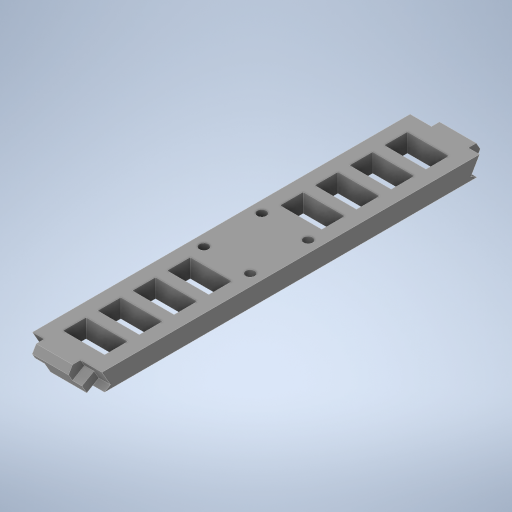
# Autodesk Inventor part: base
Saved by Autodesk Inventor 2024.3 (Build 283343000, 343)
## iProperties
Created: 2024-10-09
Part Number: base
Material: Generic
Document SubType Name: Modeling
Designer: pjcaa
Density: 1 g/cm^3
Appearance: Default(2)
Author: pjcaa
Autodesk Inventor part; units mm, degrees
ref_plane "YZ Plane" through (0, 0, 0) normal (1, 0, 0) x (0, 1, 0)
ref_plane "XZ Plane" through (0, 0, 0) normal (0, 1, 0) x (-1, 0, 0)
ref_plane "XY Plane" through (0, 0, 0) normal (0, 0, 1) x (1, 0, 0)
sketch "Sketch1" plane through (0, 0, 0) normal (0, 0, 1) x (1, 0, 0)
  line L0 (-85, -15) -> (85, -15)
  line L1 (85, -15) -> (85, 15)
  line L2 (85, 15) -> (-85, 15)
  line L3 (-85, 15) -> (-85, -15)
  line L4 (-85, -15) -> (85, 15) construction
  line L5 (85, -15) -> (-85, 15) construction
  point P0 (0, 0)
  dimension "d0" = 170
  dimension "d1" = 30
  constraints: 12 end point, 2 midpoint, 2 parallel, 1 horizontal, 1 perpendicular
  measures "d0" distance of L2.end L1.end
  measures "d1" distance of L1.end L0.end
extrude "Extrusion1" add sketch "Sketch1" along normal blind 8
sketch "Sketch2" plane through (-85, 15, 0) normal (0, 1, 0) x (1, 0, 0)
  line L0 (170, 0) -> (0, 0) construction
  line L1 (0, 0) -> (0, -8) construction
  line L2 (170, -8) -> (0, -8) construction
  line L3 (170, 0) -> (170, -8) construction
  line L4 (85, 0) -> (85, -8) construction
  line L5 (0, -8) -> (0, 0)
  line L6 (4.6188, 0) -> (0, 0)
  line L7 (4.6188, 0) -> (0, -8)
  line L8 (170, -8) -> (170, 0)
  line L9 (165.3812, 0) -> (170, 0)
  line L10 (165.3812, 0) -> (170, -8)
  dimension "d10" = 30
  constraints: 14 end point, 1 collinear, 1 midpoint, 1 perpendicular, 1 point on line, 1 symmetric about line
  measures "d10" angle of L7 L1
extrude "Extrusion3" cut sketch "Sketch2" against normal through all
sketch "Sketch3" plane through (0, 0, 8) normal (0, 0, 1) x (1, 0, 0)
  line L0 (-12.5, 10) -> (12.5, 10) construction
  line L1 (12.5, 10) -> (12.5, -10) construction
  line L2 (12.5, -10) -> (-12.5, -10) construction
  line L3 (-12.5, -10) -> (-12.5, 10) construction
  line L4 (-12.5, 10) -> (12.5, -10) construction
  line L5 (12.5, 10) -> (-12.5, -10) construction
  point P0 (0, 0)
  dimension "d11" = 25
  dimension "d12" = 20
  constraints: 12 end point, 4 coincident, 2 midpoint, 2 parallel, 1 horizontal, 1 perpendicular
  measures "d11" distance of L1.end L2.end
  measures "d12" distance of L0.end L1.end
hole "Hole1" at (-12.5, 10, 8) at (12.5, 10, 8) at (12.5, -10, 8) at (-12.5, -10, 8) direction (0, 0, -1) diameter 4 end through all
sketch "Sketch7" plane through (-85, -15, 8) normal (-0.8660254, 0, -0.5) x (-0.5, 0, 0.8660254)
  line L0 (0, 0) -> (-9.2376, 0) construction
  line L1 (0, 30) -> (0, 0) construction
  line L2 (-9.2376, 30) -> (0, 30) construction
  line L3 (-9.2376, 0) -> (-9.2376, 30) construction
  line L4 (0, 30) -> (-9.2376, 30)
  line L5 (-9.2376, 30) -> (-9.2376, 20.7624)
  line L6 (-9.2376, 20.7624) -> (-4.1376, 20.7624)
  line L7 (-4.1376, 20.7624) -> (-4.1376, 24.9)
  line L8 (-4.1376, 24.9) -> (0, 24.9)
  line L9 (0, 24.9) -> (0, 30)
  line L10 (0, 0) -> (0, 9.2376)
  line L11 (0, 9.2376) -> (-5.1, 9.2376)
  line L12 (-5.1, 9.2376) -> (-5.1, 5.1)
  line L13 (-5.1, 5.1) -> (-9.2376, 5.1)
  line L14 (-9.2376, 5.1) -> (-9.2376, 0)
  line L15 (-9.2376, 0) -> (0, 0)
  point P0 (-49.4282, 15)
  dimension "d30" = 5.1
  dimension "d31" = 5.1
  dimension "d32" = 5.1
  constraints: 24 end point, 6 perpendicular, 4 point on line, 3 equal length, 2 collinear, 2 horizontal
  measures "d30" distance of L5.end L6.end
  measures "d31" distance between parallel lines of L8 L2
  measures "d32" distance between parallel lines of L0 L13
extrude "Extrusion7" cut sketch "Sketch7" against normal blind 3
sketch "Sketch8" plane through (-85, -5.7624, 8) normal (-0.8660254, 0, -0.5) x (-0.5, 0, 0.8660254)
  line L0 (-5.1, 0) -> (0, 0) projected
  line L1 (0, 15.6624) -> (0, 0) projected
  line L2 (0, 15.6624) -> (-4.1376, 15.6624) projected
  line L3 (-4.1376, 15.6624) -> (-4.1376, 11.5248) projected
  line L4 (-4.1376, 11.5248) -> (-9.2376, 11.5248) projected
  line L5 (-9.2376, -4.1376) -> (-9.2376, 11.5248) projected
  line L6 (-9.2376, -4.1376) -> (-5.1, -4.1376) projected
  line L7 (-5.1, -4.1376) -> (-5.1, 0) projected
  point P0 (-49.4282, 5.7624)
extrude "Extrusion8" add sketch "Sketch8" along normal blind 3
sketch "Sketch10" plane through (80.3812, -15, 0) normal (0.8660254, 0, -0.5) x (-0.5, 0, -0.8660254)
  line L0 (0, 0) -> (-9.2376, 0) construction
  line L1 (0, 30) -> (0, 0) construction
  line L2 (-9.2376, 30) -> (0, 30) construction
  line L3 (-9.2376, 0) -> (-9.2376, 30) construction
  line L4 (-9.2376, 0) -> (0, 0)
  line L5 (0, 0) -> (0, 9.2376)
  line L6 (0, 9.2376) -> (-4.9, 9.2376)
  line L7 (-4.9, 9.2376) -> (-4.9, 4.9)
  line L8 (-4.9, 4.9) -> (-9.2376, 4.9)
  line L9 (-9.2376, 4.9) -> (-9.2376, 0)
  line L10 (-9.2376, 30) -> (-9.2376, 20.7624)
  line L11 (-9.2376, 20.7624) -> (-4.3376, 20.7624)
  line L12 (-4.3376, 20.7624) -> (-4.3376, 25.1)
  line L13 (-4.3376, 25.1) -> (0, 25.1)
  line L14 (0, 25.1) -> (0, 30)
  line L15 (0, 30) -> (-9.2376, 30)
  point P0 (40.1906, 15)
  point P1 (-2.1688, 25.1)
  dimension "d40" = 4.9
  dimension "d41" = 4.9
  dimension "d42" = 4.9
  constraints: 24 end point, 5 perpendicular, 4 point on line, 3 equal length, 3 horizontal, 2 collinear, 1 midpoint
  measures "d40" distance between parallel lines of L0 L8
  measures "d41" distance of L5.end L6.end
  measures "d42" distance from line of point (-2.169, 25.1) L2
extrude "Extrusion10" cut sketch "Sketch10" against normal blind 3
sketch "Sketch11" plane through (85, -10.1, 8) normal (0.8660254, 0, -0.5) x (-0.5, 0, -0.8660254)
  line L0 (4.9, 15.8624) -> (0, 15.8624) projected
  line L1 (0, 0) -> (0, 15.8624) projected
  line L2 (0, 0) -> (4.3376, 0) projected
  line L3 (4.3376, 0) -> (4.3376, 4.3376) projected
  line L4 (4.3376, 4.3376) -> (9.2376, 4.3376) projected
  line L5 (9.2376, 20.2) -> (9.2376, 4.3376) projected
  line L6 (9.2376, 20.2) -> (4.9, 20.2) projected
  line L7 (4.9, 20.2) -> (4.9, 15.8624) projected
  point P0 (49.4282, 10.1)
extrude "Extrusion11" add sketch "Sketch11" along normal blind 3
sketch "Sketch9" plane through (-80.3812, -15, 0) normal (0, -1, 0) x (1, 0, 0)
  line L0 (-4.6188, 8) -> (-1.1547, 8) construction
  line L1 (-4.6188, 8) -> (-7.2169, 6.5) construction
  line L2 (-4.6669, 2.0833) -> (-7.2169, 6.5) construction
  line L3 (0.5293, 5.0833) -> (-4.6669, 2.0833) construction
  line L4 (0.5293, 5.0833) -> (-1.1547, 8) construction
  line L5 (-4.6188, 8) -> (-7.2169, 6.5)
  line L6 (-7.2169, 6.5) -> (-6.3509, 5)
  line L7 (-6.3509, 5) -> (-4.6188, 8)
  line L8 (161.9171, 8) -> (165.3812, 8) construction
  line L9 (161.9171, 8) -> (160.6143, 5.7435) construction
  line L10 (165.8105, 2.7435) -> (160.6143, 5.7435) construction
  line L11 (167.9793, 6.5) -> (165.8105, 2.7435) construction
  line L12 (165.3812, 8) -> (167.9793, 6.5) construction
  line L13 (167.9793, 6.5) -> (167.1132, 5)
  line L14 (167.1132, 5) -> (165.3812, 8)
  line L15 (167.9793, 6.5) -> (165.3812, 8)
  point P0 (80.3812, 0)
  dimension "d37" = 30
  dimension "d47" = 30
  constraints: 12 end point, 3 point on line, 1 collinear
  measures "d37" angle of L1 L7
  measures "d47" angle of L12 L14
extrude "Extrusion9" cut sketch "Sketch9" against normal through all
sketch "Sketch12" plane through (0, 0, 0) normal (0, 0, -1) x (-1, 0, 0)
  circle A0 centre (12.5, -10) radius 2 construction
  circle A1 centre (-12.5, -10) radius 2 construction
  circle A2 centre (-12.5, 10) radius 2 construction
  circle A3 centre (12.5, 10) radius 2 construction
  line L0 (-80.3812, 15) -> (-80.3812, 10.1) construction
  line L1 (-80.3812, 10.1) -> (-80.3812, -5.7624) construction
  line L2 (-80.3812, -5.7624) -> (-80.3812, -15) construction
  line L3 (80.3812, -15) -> (-80.3812, -15) construction
  line L4 (80.3812, -15) -> (80.3812, -9.9) construction
  line L5 (80.3812, -9.9) -> (80.3812, 5.7624) construction
  line L6 (80.3812, 5.7624) -> (80.3812, 15) construction
  line L7 (-80.3812, 15) -> (80.3812, 15) construction
  line L8 (0, -15) -> (0, 15) construction
  line L9 (74.3812, -9) -> (64.3812, -9)
  line L10 (64.3812, -9) -> (64.3812, 9)
  line L11 (64.3812, 9) -> (74.3812, 9)
  line L12 (74.3812, 9) -> (74.3812, -9)
  line L13 (49.3812, -9) -> (49.3812, 9)
  line L14 (59.3812, -9) -> (49.3812, -9)
  line L15 (49.3812, 9) -> (59.3812, 9)
  line L16 (59.3812, 9) -> (59.3812, -9)
  line L17 (34.3812, -9) -> (34.3812, 9)
  line L18 (44.3812, -9) -> (34.3812, -9)
  line L19 (34.3812, 9) -> (44.3812, 9)
  line L20 (44.3812, 9) -> (44.3812, -9)
  line L21 (19.3812, -9) -> (19.3812, 9)
  line L22 (29.3812, -9) -> (19.3812, -9)
  line L23 (19.3812, 9) -> (29.3812, 9)
  line L24 (29.3812, 9) -> (29.3812, -9)
  line L25 (-74.3812, -9) -> (-64.3812, -9)
  line L26 (-64.3812, -9) -> (-64.3812, 9)
  line L27 (-64.3812, 9) -> (-74.3812, 9)
  line L28 (-74.3812, 9) -> (-74.3812, -9)
  line L29 (-49.3812, -9) -> (-49.3812, 9)
  line L30 (-59.3812, -9) -> (-49.3812, -9)
  line L31 (-49.3812, 9) -> (-59.3812, 9)
  line L32 (-59.3812, 9) -> (-59.3812, -9)
  line L33 (-34.3812, -9) -> (-34.3812, 9)
  line L34 (-44.3812, -9) -> (-34.3812, -9)
  line L35 (-34.3812, 9) -> (-44.3812, 9)
  line L36 (-44.3812, 9) -> (-44.3812, -9)
  line L37 (-19.3812, -9) -> (-19.3812, 9)
  line L38 (-29.3812, -9) -> (-19.3812, -9)
  line L39 (-19.3812, 9) -> (-29.3812, 9)
  line L40 (-29.3812, 9) -> (-29.3812, -9)
  point P0 (0, 0)
  point P1 (0, 0)
  point P2 (64.3812, 0)
  point P3 (49.3812, 0)
  point P4 (34.3812, 0)
  point P5 (19.3812, 0)
  point P6 (-64.3812, 0)
  point P7 (-49.3812, 0)
  point P8 (-34.3812, 0)
  point P9 (-19.3812, 0)
  dimension "d48" = 10
  dimension "d49" = 18
  dimension "d50" = 6
  dimension "d53" = 15
  constraints: 66 end point, 20 symmetric about line, 4 midpoint, 2 horizontal, 2 parallel, 1 horizontal alignment, 1 perpendicular, 27 other
  measures "d48" distance of L10.end L11.end
  measures "d49" distance of L9.end L10.end
  measures "d50" horizontal distance of L3.start L9.start
  measures "d53" distance of L10.end L13.end
extrude "Extrusion12" cut sketch "Sketch12" against normal through all
body "Solid1"
